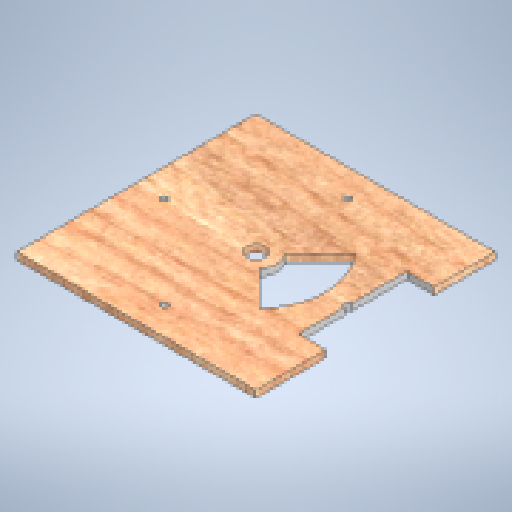
# Autodesk Inventor part: Plataforma
Saved by Autodesk Inventor 2023 (Build 270158000, 158)
## iProperties
Created: 2022-11-24
Part Number: Plataforma
Material: Genérico
Document SubType Name: Modeling
Designer: sergi
Density: 1 g/cm^3
Appearance: Valor por defecto
Author: sergi
Autodesk Inventor part; units mm, degrees
ref_plane "YZ Plane" through (0, 0, 0) normal (1, 0, 0) x (0, 1, 0)
ref_plane "XZ Plane" through (0, 0, 0) normal (0, 1, 0) x (-1, 0, 0)
ref_plane "XY Plane" through (0, 0, 0) normal (0, 0, 1) x (1, 0, 0)
sketch "Boceto6" plane through (0, 0, 0) normal (0, 1, 0) x (-1, 0, 0)
  line L0 (-51.5, -51.5) -> (51.5, -51.5)
  line L1 (51.5, -51.5) -> (51.5, 51.5)
  line L2 (51.5, 51.5) -> (-51.5, 51.5)
  line L3 (-51.5, 51.5) -> (-51.5, -51.5)
  line L4 (-53.9142, 52.5) -> (52.5, 52.5)
  line L5 (52.5, 52.5) -> (52.5, -53.9142)
  line L6 (52.5, 53.9142) -> (52.5, -52.5)
  line L7 (52.5, -52.5) -> (-53.9142, -52.5)
  arc A0 (-21.9085, 20.4943) -> (-21.9085, -20.4943) centre (0, 0) ccw
  line L8 (-53.9142, -52.5) -> (-51.5, -50.0858)
  line L9 (-21.9085, -20.4943) -> (-7.0317, -5.6174)
  line L10 (-7.0317, 5.6174) -> (-21.9085, 20.4943)
  line L11 (-51.5, 50.0858) -> (-53.9142, 52.5)
  circle A1 centre (0, 0) radius 4.1
  arc A2 (-7.0317, 5.6174) -> (-7.0317, -5.6174) centre (0, 0) ccw
  dimension "d32" = 103
  dimension "d33" = 103
  dimension "d39" = 8.2
  dimension "d49" = 18
  constraints: 24 end point, 4 point on circle, 3 centre point, 2 parallel, 2 perpendicular, 2 point on line, 1 coincident, 1 horizontal, 2 other
  measures "d32" distance of L2.end L1.end
  measures "d33" distance of L1.end L0.end
  measures "d39" diameter of A1
  measures "d49" diameter of A2
extrude "Extrusión4" add sketch "Boceto6" along normal blind 3 contours L3 L2 L1 L0
sketch "Boceto7" plane through (0, 3, 0) normal (0, 1, 0) x (1, 0, 0)
  circle A0 centre (39.5, 0) radius 1.5 projected
  circle A1 centre (0, 39.5) radius 1.5 projected
  line L0 (51.5, -51.5) -> (51.5, 51.5) projected
  line L1 (-51.5, -51.5) -> (51.5, -51.5) projected
  line L2 (-51.5, 51.5) -> (-51.5, -51.5) projected
  line L3 (51.5, 51.5) -> (-51.5, 51.5) projected
  arc A2 (-5.9631, 4.5488) -> (-5.9631, -4.5488) centre (0, 0) ccw projected
  line L4 (-21.9085, 20.4943) -> (-5.9631, 4.5488) projected
  arc A3 (-21.9085, 20.4943) -> (-21.9085, -20.4943) centre (0, 0) ccw projected
  line L5 (-5.9631, -4.5488) -> (-21.9085, -20.4943) projected
  circle A4 centre (-39.5, 0) radius 1.5 projected
  circle A5 centre (0, -39.5) radius 1.5 projected
  point P0 (0, 0)
hole "Agujero3" at (39.5, 3, 0) at (0, 3, -39.5) at (-39.5, 3, 0) at (0, 3, 39.5) direction (0, -1, 0) diameter 3 end through all
sketch "Boceto8" plane through (0, 3, 0) normal (0, 1, 0) x (1, 0, 0)
  line L0 (51.5, -51.5) -> (51.5, -21.5)
  line L1 (51.5, -51.5) -> (51.5, 51.5) projected
  line L2 (51.5, -21.5) -> (39.7367, -21.5)
  line L3 (39.7367, -21.5) -> (39.7367, 25.2431)
  line L4 (39.7367, 25.2431) -> (51.5, 25.2431)
  line L5 (51.5, 25.2431) -> (51.5, -21.5)
  point P0 (0, 0)
  dimension "d50" = 30
  constraints: 10 end point, 2 parallel, 1 horizontal, 1 perpendicular, 1 point on line
  measures "d50" distance of L0.start L0.end
extrude "Extrusión5" cut sketch "Boceto8" against normal blind 10
